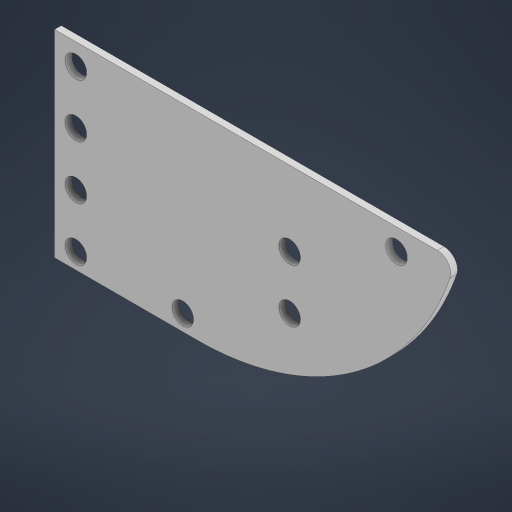
# Autodesk Inventor part: Sleds
Saved by Autodesk Inventor 2023.4 (Build 274418000, 418)
## iProperties
Created: 2023-12-10
Part Number: Sleds
Material: Generic
Document SubType Name: Modeling
Designer: diego
Density: 1 g/cm^3
Appearance: Default
Author: diego
Autodesk Inventor part; units mm, degrees
ref_plane "YZ Plane" through (0, 0, 0) normal (1, 0, 0) x (0, 1, 0)
ref_plane "XZ Plane" through (0, 0, 0) normal (0, 1, 0) x (-1, 0, 0)
ref_plane "XY Plane" through (0, 0, 0) normal (0, 0, 1) x (1, 0, 0)
sketch "Sketch1" plane through (0, 0, 0) normal (0, 0, 1) x (1, 0, 0)
  circle A0 centre (0, 0) radius 63.5
  line L0 (0, 0) -> (63.5, 0)
  line L1 (0, 0) -> (0, -63.5)
  line L2 (0, 0) -> (-127, 0)
  line L3 (-127, 0) -> (-127, -63.5)
  line L4 (-127, -63.5) -> (0, -63.5)
  line L5 (-127, 0) -> (-127, -16.51)
  line L6 (-127, -16.51) -> (61.3161, -16.51)
  dimension "d0" = 127
  dimension "d1" = 127
  dimension "d43" = 16.51
  constraints: 14 end point, 4 perpendicular, 3 point on circle, 1 centre point, 1 coincident, 1 point on line, 1 tangent, 1 vertical
  measures "d0" diameter of A0
  measures "d1" distance of L0.start L2.end
  measures "d43" distance of L2.end L5.end
extrude "Extrusion4" add sketch "Sketch1" along normal blind 1.5875 contours L1 L6 A0 | L4 L3 L6 A0 | A0 L6 L1
sketch "Sketch4" plane through (0, 0, 1.5875) normal (0, 0, 1) x (1, 0, 0)
  arc A0 (0, -63.5) -> (61.3161, -16.51) centre (0, 0) ccw projected
  line L0 (61.3161, -16.51) -> (-59.3339, -16.51)
  line L1 (61.3161, -16.51) -> (-127, -16.51) projected
  line L2 (-59.3339, -16.51) -> (-59.3339, -62.6422)
  line L3 (-59.3339, -62.6422) -> (-59.3339, -63.5)
  line L4 (-127, -63.5) -> (0, -63.5) projected
  line L5 (-136.3806, -11.9346) -> (-59.3339, -11.9346)
  line L6 (-59.3339, -11.9346) -> (-59.3339, -68.0966)
  line L7 (-59.3339, -68.0966) -> (-136.3806, -68.0966)
  line L8 (-136.3806, -68.0966) -> (-136.3806, -11.9346)
  point P0 (-59.3339, -16.51)
  dimension "d46" = 120.65
  constraints: 14 end point, 3 point on line, 2 parallel, 2 perpendicular, 1 horizontal
  measures "d46" distance of L0.start L0.end
extrude "Extrusion5" cut sketch "Sketch4" against normal blind 1.5875 contours L6 L7 L8 L5 L2 L3
fillet "Fillet2" radius 3.175 1 edges at (61.3161, -16.51, 0.7937)
fillet "Fillet3" radius 3.175 2 edges at (-59.3339, -63.5, 0.7937) (-59.3339, -16.51, 0.7937)
sketch "Sketch5" plane through (0, 0, 1.5875) normal (0, 0, 1) x (1, 0, 0)
  circle A0 centre (-55.6881, -20.1151) radius 2.54
  line L0 (-55.6881, -20.1151) -> (-55.6881, -45.5151)
  line L1 (-55.6881, -45.5151) -> (-55.6881, -58.2151)
  circle A1 centre (-55.6881, -58.2151) radius 2.54
  line L2 (-55.6881, -20.1151) -> (-30.2881, -20.1151)
  line L3 (-55.6881, -58.2151) -> (-30.2881, -58.2151)
  circle A2 centre (-55.6881, -45.5151) radius 2.54
  circle A3 centre (-55.6881, -32.8151) radius 2.54
  line L4 (-59.3339, -13.3218) -> (-33.9321, -13.3218)
  line L5 (-33.9321, -13.3218) -> (-33.9321, -67.3178)
  line L6 (-33.9321, -67.3178) -> (-59.3339, -67.3178)
  line L7 (-59.3339, -67.3178) -> (-59.3339, -13.3218)
  point P0 (0, 0)
  point P1 (-4.8881, -58.2151)
  point P2 (7.8119, -58.2151)
  point P3 (-59.3339, -20.1151)
  point P4 (-42.9881, -20.1151)
  point P5 (-42.9881, -58.2151)
  dimension "d51" = 5.08
  dimension "d52" = 25.4
  dimension "d53" = 12.7
  dimension "d54" = 5.08
  dimension "d55" = 25.4
  dimension "d63" = 25.4
  dimension "d68" = 5.08
  dimension "d69" = 5.08
  constraints: 16 end point, 5 midpoint, 4 centre point, 4 coincident, 3 horizontal, 2 parallel, 2 vertical, 1 perpendicular
  measures "d51" diameter of A0
  measures "d52" distance of L0.start L0.end
  measures "d53" distance of L0.end L1.end
  measures "d54" diameter of A1
  measures "d55" distance of L0.start L2.end
  measures "d63" distance of L3.start L3.end
  measures "d68" diameter of A2
  measures "d69" diameter of A3
extrude "Extrusion6" cut sketch "Sketch5" against normal blind 1.5875
sketch "Sketch6" plane through (0, 0, 1.5875) normal (0, 0, 1) x (1, 0, 0)
  line L0 (57.0229, -16.51) -> (-33.9321, -16.51) projected
  line L1 (-33.9321, -63.5) -> (-33.9321, -16.51) projected
  line L2 (-33.9321, -21.59) -> (-33.9321, -26.67)
  line L3 (-33.9321, -21.59) -> (-28.8521, -21.59)
  line L4 (-28.8521, -21.59) -> (-28.8521, -16.51)
  circle A0 centre (-28.8521, -21.59) radius 2.54
  line L5 (-28.8521, -21.59) -> (-28.8521, -46.99)
  line L6 (-28.8521, -46.99) -> (-28.8521, -59.69)
  circle A1 centre (-28.8521, -59.69) radius 2.54
  line L7 (-28.8521, -21.59) -> (-3.4521, -21.59)
  line L8 (-3.4521, -21.59) -> (21.9479, -21.59)
  line L9 (21.9479, -21.59) -> (47.3479, -21.59)
  circle A2 centre (-28.8521, -34.29) radius 2.54
  circle A3 centre (-28.8521, -46.99) radius 2.54
  line L10 (-28.8521, -59.69) -> (-3.4521, -59.69)
  line L11 (-3.4521, -59.69) -> (9.2479, -59.69)
  circle A4 centre (-3.4521, -59.69) radius 2.54
  circle A5 centre (47.3479, -21.59) radius 2.54
  line L12 (21.9479, -34.29) -> (21.9479, -46.99)
  circle A6 centre (21.9479, -34.29) radius 2.54
  circle A7 centre (21.9479, -46.99) radius 2.54
  point P0 (0, 0)
  dimension "d80" = 5.08
  dimension "d81" = 5.08
  dimension "d82" = 5.08
  dimension "d83" = 25.4
  dimension "d84" = 12.7
  dimension "d85" = 5.08
  dimension "d86" = 25.4
  dimension "d87" = 25.4
  dimension "d88" = 25.4
  dimension "d89" = 5.08
  dimension "d90" = 5.08
  dimension "d91" = 25.4
  dimension "d92" = 12.7
  dimension "d93" = 5.08
  dimension "d96" = 5.08
  dimension "d99" = 5.08
  dimension "d100" = 5.08
  constraints: 22 end point, 10 coincident, 8 centre point, 5 point on line, 4 horizontal, 1 midpoint, 1 perpendicular, 1 vertical
  measures "d80" distance of L2.start L2.end
  measures "d81" distance of L2.start L3.end
  measures "d82" diameter of A0
  measures "d83" distance of L5.start L5.end
  measures "d84" distance of L5.end L6.end
  measures "d85" diameter of A1
  measures "d86" distance of L5.start L7.end
  measures "d87" distance of L8.start L8.end
  measures "d88" distance of L9.start L9.end
  measures "d89" diameter of A2
  measures "d90" diameter of A3
  measures "d91" distance of L10.start L10.end
  measures "d92" distance of L10.end L11.end
  measures "d93" diameter of A4
  measures "d96" diameter of A5
  measures "d99" diameter of A6
  measures "d100" diameter of A7
extrude "Extrusion7" cut sketch "Sketch6" against normal blind 5.08 contours A0 L7 L4 | L4 L3 A0 | L5 A0 L3 | L7 A0 L5 | A2 L5 | L5 A2 | A3 L6 L5 | L5 L6 A3 | A1 L10 L6 | L6 L10 A1 | A4 L11 L10 | L10 L11 A4 | A5 | A6 | A7
equation "\"d97\" = d93"
body "Solid1"
